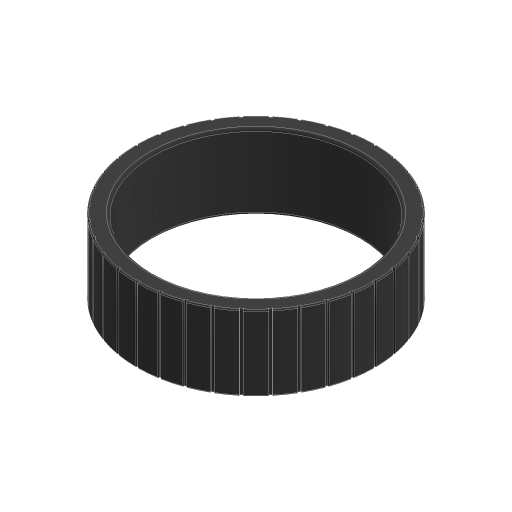
# Autodesk Inventor part: rubber
Saved by Autodesk Inventor 2023 (Build 270158000, 158)
## iProperties
Created: 2022-09-21
Part Number: rubber
Material: 고무
Document SubType Name: Modeling
Designer: doore
Density: 0.93 g/cm^3
Appearance: 고무 - 검은색
Author: doore
Autodesk Inventor part; units mm, degrees
ref_plane "YZ Plane" through (0, 0, 0) normal (1, 0, 0) x (0, 1, 0)
ref_plane "XZ Plane" through (0, 0, 0) normal (0, 1, 0) x (-1, 0, 0)
ref_plane "XY Plane" through (0, 0, 0) normal (0, 0, 1) x (1, 0, 0)
sketch "스케치1" plane through (0, 0, 0) normal (0, 1, 0) x (-1, 0, 0)
  circle A0 centre (0, 0) radius 27.5
  circle A1 centre (0, 0) radius 31.8
  line L0 (-31.25, -0.35) -> (-32.35, -0.35)
  line L1 (-32.35, -0.35) -> (-32.35, 0.35)
  line L2 (-32.35, 0.35) -> (-31.25, 0.35)
  line L3 (-31.25, 0.35) -> (-31.25, -0.35)
  circle A2 centre (0, 0) radius 31.8
  line L4 (-31.25, -0.35) -> (-32.35, 0.35) construction
  line L5 (-32.35, -0.35) -> (-31.25, 0.35) construction
  line L6 (-30.7145, -5.7712) -> (-31.7978, -5.9622)
  line L7 (-31.7978, -5.9622) -> (-31.9193, -5.2728)
  line L8 (-31.9193, -5.2728) -> (-30.836, -5.0818)
  line L9 (-30.836, -5.0818) -> (-30.7145, -5.7712)
  line L10 (-30.7145, -5.7712) -> (-31.9193, -5.2728) construction
  line L11 (-31.7978, -5.9622) -> (-30.836, -5.0818) construction
  line L12 (-29.2457, -11.017) -> (-30.2793, -11.3932)
  line L13 (-30.2793, -11.3932) -> (-30.5188, -10.7355)
  line L14 (-30.5188, -10.7355) -> (-29.4851, -10.3592)
  line L15 (-29.4851, -10.3592) -> (-29.2457, -11.017)
  line L16 (-29.2457, -11.017) -> (-30.5188, -10.7355) construction
  line L17 (-30.2793, -11.3932) -> (-29.4851, -10.3592) construction
  line L18 (-26.8883, -15.9281) -> (-27.8409, -16.4781)
  line L19 (-27.8409, -16.4781) -> (-28.1909, -15.8719)
  line L20 (-28.1909, -15.8719) -> (-27.2383, -15.3219)
  line L21 (-27.2383, -15.3219) -> (-26.8883, -15.9281)
  line L22 (-26.8883, -15.9281) -> (-28.1909, -15.8719) construction
  line L23 (-27.8409, -16.4781) -> (-27.2383, -15.3219) construction
  line L24 (-23.7139, -20.3552) -> (-24.5566, -21.0623)
  line L25 (-24.5566, -21.0623) -> (-25.0065, -20.5261)
  line L26 (-25.0065, -20.5261) -> (-24.1639, -19.819)
  line L27 (-24.1639, -19.819) -> (-23.7139, -20.3552)
  line L28 (-23.7139, -20.3552) -> (-25.0065, -20.5261) construction
  line L29 (-24.5566, -21.0623) -> (-24.1639, -19.819) construction
  line L30 (-19.819, -24.1639) -> (-20.5261, -25.0065)
  line L31 (-20.5261, -25.0065) -> (-21.0623, -24.5566)
  line L32 (-21.0623, -24.5566) -> (-20.3552, -23.7139)
  line L33 (-20.3552, -23.7139) -> (-19.819, -24.1639)
  line L34 (-19.819, -24.1639) -> (-21.0623, -24.5566) construction
  line L35 (-20.5261, -25.0065) -> (-20.3552, -23.7139) construction
  line L36 (-15.3219, -27.2383) -> (-15.8719, -28.1909)
  line L37 (-15.8719, -28.1909) -> (-16.4781, -27.8409)
  line L38 (-16.4781, -27.8409) -> (-15.9281, -26.8883)
  line L39 (-15.9281, -26.8883) -> (-15.3219, -27.2383)
  line L40 (-15.3219, -27.2383) -> (-16.4781, -27.8409) construction
  line L41 (-15.8719, -28.1909) -> (-15.9281, -26.8883) construction
  line L42 (-10.3592, -29.4851) -> (-10.7355, -30.5188)
  line L43 (-10.7355, -30.5188) -> (-11.3932, -30.2793)
  line L44 (-11.3932, -30.2793) -> (-11.017, -29.2457)
  line L45 (-11.017, -29.2457) -> (-10.3592, -29.4851)
  line L46 (-10.3592, -29.4851) -> (-11.3932, -30.2793) construction
  line L47 (-10.7355, -30.5188) -> (-11.017, -29.2457) construction
  line L48 (-5.0818, -30.836) -> (-5.2728, -31.9193)
  line L49 (-5.2728, -31.9193) -> (-5.9622, -31.7978)
  line L50 (-5.9622, -31.7978) -> (-5.7712, -30.7145)
  line L51 (-5.7712, -30.7145) -> (-5.0818, -30.836)
  line L52 (-5.0818, -30.836) -> (-5.9622, -31.7978) construction
  line L53 (-5.2728, -31.9193) -> (-5.7712, -30.7145) construction
  line L54 (0.35, -31.25) -> (0.35, -32.35)
  line L55 (0.35, -32.35) -> (-0.35, -32.35)
  line L56 (-0.35, -32.35) -> (-0.35, -31.25)
  line L57 (-0.35, -31.25) -> (0.35, -31.25)
  line L58 (0.35, -31.25) -> (-0.35, -32.35) construction
  line L59 (0.35, -32.35) -> (-0.35, -31.25) construction
  line L60 (5.7712, -30.7145) -> (5.9622, -31.7978)
  line L61 (5.9622, -31.7978) -> (5.2728, -31.9193)
  line L62 (5.2728, -31.9193) -> (5.0818, -30.836)
  line L63 (5.0818, -30.836) -> (5.7712, -30.7145)
  line L64 (5.7712, -30.7145) -> (5.2728, -31.9193) construction
  line L65 (5.9622, -31.7978) -> (5.0818, -30.836) construction
  line L66 (11.017, -29.2457) -> (11.3932, -30.2793)
  line L67 (11.3932, -30.2793) -> (10.7355, -30.5188)
  line L68 (10.7355, -30.5188) -> (10.3592, -29.4851)
  line L69 (10.3592, -29.4851) -> (11.017, -29.2457)
  line L70 (11.017, -29.2457) -> (10.7355, -30.5188) construction
  line L71 (11.3932, -30.2793) -> (10.3592, -29.4851) construction
  line L72 (15.9281, -26.8883) -> (16.4781, -27.8409)
  line L73 (16.4781, -27.8409) -> (15.8719, -28.1909)
  line L74 (15.8719, -28.1909) -> (15.3219, -27.2383)
  line L75 (15.3219, -27.2383) -> (15.9281, -26.8883)
  line L76 (15.9281, -26.8883) -> (15.8719, -28.1909) construction
  line L77 (16.4781, -27.8409) -> (15.3219, -27.2383) construction
  line L78 (20.3552, -23.7139) -> (21.0623, -24.5566)
  line L79 (21.0623, -24.5566) -> (20.5261, -25.0065)
  line L80 (20.5261, -25.0065) -> (19.819, -24.1639)
  line L81 (19.819, -24.1639) -> (20.3552, -23.7139)
  line L82 (20.3552, -23.7139) -> (20.5261, -25.0065) construction
  line L83 (21.0623, -24.5566) -> (19.819, -24.1639) construction
  line L84 (24.1639, -19.819) -> (25.0065, -20.5261)
  line L85 (25.0065, -20.5261) -> (24.5566, -21.0623)
  line L86 (24.5566, -21.0623) -> (23.7139, -20.3552)
  line L87 (23.7139, -20.3552) -> (24.1639, -19.819)
  line L88 (24.1639, -19.819) -> (24.5566, -21.0623) construction
  line L89 (25.0065, -20.5261) -> (23.7139, -20.3552) construction
  line L90 (27.2383, -15.3219) -> (28.1909, -15.8719)
  line L91 (28.1909, -15.8719) -> (27.8409, -16.4781)
  line L92 (27.8409, -16.4781) -> (26.8883, -15.9281)
  line L93 (26.8883, -15.9281) -> (27.2383, -15.3219)
  line L94 (27.2383, -15.3219) -> (27.8409, -16.4781) construction
  line L95 (28.1909, -15.8719) -> (26.8883, -15.9281) construction
  line L96 (29.4851, -10.3592) -> (30.5188, -10.7355)
  line L97 (30.5188, -10.7355) -> (30.2793, -11.3932)
  line L98 (30.2793, -11.3932) -> (29.2457, -11.017)
  line L99 (29.2457, -11.017) -> (29.4851, -10.3592)
  line L100 (29.4851, -10.3592) -> (30.2793, -11.3932) construction
  line L101 (30.5188, -10.7355) -> (29.2457, -11.017) construction
  line L102 (30.836, -5.0818) -> (31.9193, -5.2728)
  line L103 (31.9193, -5.2728) -> (31.7978, -5.9622)
  line L104 (31.7978, -5.9622) -> (30.7145, -5.7712)
  line L105 (30.7145, -5.7712) -> (30.836, -5.0818)
  line L106 (30.836, -5.0818) -> (31.7978, -5.9622) construction
  line L107 (31.9193, -5.2728) -> (30.7145, -5.7712) construction
  line L108 (31.25, 0.35) -> (32.35, 0.35)
  line L109 (32.35, 0.35) -> (32.35, -0.35)
  line L110 (32.35, -0.35) -> (31.25, -0.35)
  line L111 (31.25, -0.35) -> (31.25, 0.35)
  line L112 (31.25, 0.35) -> (32.35, -0.35) construction
  line L113 (32.35, 0.35) -> (31.25, -0.35) construction
  line L114 (30.7145, 5.7712) -> (31.7978, 5.9622)
  line L115 (31.7978, 5.9622) -> (31.9193, 5.2728)
  line L116 (31.9193, 5.2728) -> (30.836, 5.0818)
  line L117 (30.836, 5.0818) -> (30.7145, 5.7712)
  line L118 (30.7145, 5.7712) -> (31.9193, 5.2728) construction
  line L119 (31.7978, 5.9622) -> (30.836, 5.0818) construction
  line L120 (29.2457, 11.017) -> (30.2793, 11.3932)
  line L121 (30.2793, 11.3932) -> (30.5188, 10.7355)
  line L122 (30.5188, 10.7355) -> (29.4851, 10.3592)
  line L123 (29.4851, 10.3592) -> (29.2457, 11.017)
  line L124 (29.2457, 11.017) -> (30.5188, 10.7355) construction
  line L125 (30.2793, 11.3932) -> (29.4851, 10.3592) construction
  line L126 (26.8883, 15.9281) -> (27.8409, 16.4781)
  line L127 (27.8409, 16.4781) -> (28.1909, 15.8719)
  line L128 (28.1909, 15.8719) -> (27.2383, 15.3219)
  line L129 (27.2383, 15.3219) -> (26.8883, 15.9281)
  line L130 (26.8883, 15.9281) -> (28.1909, 15.8719) construction
  line L131 (27.8409, 16.4781) -> (27.2383, 15.3219) construction
  line L132 (23.7139, 20.3552) -> (24.5566, 21.0623)
  line L133 (24.5566, 21.0623) -> (25.0065, 20.5261)
  line L134 (25.0065, 20.5261) -> (24.1639, 19.819)
  line L135 (24.1639, 19.819) -> (23.7139, 20.3552)
  line L136 (23.7139, 20.3552) -> (25.0065, 20.5261) construction
  line L137 (24.5566, 21.0623) -> (24.1639, 19.819) construction
  line L138 (19.819, 24.1639) -> (20.5261, 25.0065)
  line L139 (20.5261, 25.0065) -> (21.0623, 24.5566)
  line L140 (21.0623, 24.5566) -> (20.3552, 23.7139)
  line L141 (20.3552, 23.7139) -> (19.819, 24.1639)
  line L142 (19.819, 24.1639) -> (21.0623, 24.5566) construction
  line L143 (20.5261, 25.0065) -> (20.3552, 23.7139) construction
  line L144 (15.3219, 27.2383) -> (15.8719, 28.1909)
  line L145 (15.8719, 28.1909) -> (16.4781, 27.8409)
  line L146 (16.4781, 27.8409) -> (15.9281, 26.8883)
  line L147 (15.9281, 26.8883) -> (15.3219, 27.2383)
  line L148 (15.3219, 27.2383) -> (16.4781, 27.8409) construction
  line L149 (15.8719, 28.1909) -> (15.9281, 26.8883) construction
  line L150 (10.3592, 29.4851) -> (10.7355, 30.5188)
  line L151 (10.7355, 30.5188) -> (11.3932, 30.2793)
  line L152 (11.3932, 30.2793) -> (11.017, 29.2457)
  line L153 (11.017, 29.2457) -> (10.3592, 29.4851)
  line L154 (10.3592, 29.4851) -> (11.3932, 30.2793) construction
  line L155 (10.7355, 30.5188) -> (11.017, 29.2457) construction
  line L156 (5.0818, 30.836) -> (5.2728, 31.9193)
  line L157 (5.2728, 31.9193) -> (5.9622, 31.7978)
  line L158 (5.9622, 31.7978) -> (5.7712, 30.7145)
  line L159 (5.7712, 30.7145) -> (5.0818, 30.836)
  line L160 (5.0818, 30.836) -> (5.9622, 31.7978) construction
  line L161 (5.2728, 31.9193) -> (5.7712, 30.7145) construction
  line L162 (-0.35, 31.25) -> (-0.35, 32.35)
  line L163 (-0.35, 32.35) -> (0.35, 32.35)
  line L164 (0.35, 32.35) -> (0.35, 31.25)
  line L165 (0.35, 31.25) -> (-0.35, 31.25)
  line L166 (-0.35, 31.25) -> (0.35, 32.35) construction
  line L167 (-0.35, 32.35) -> (0.35, 31.25) construction
  line L168 (-5.7712, 30.7145) -> (-5.9622, 31.7978)
  line L169 (-5.9622, 31.7978) -> (-5.2728, 31.9193)
  line L170 (-5.2728, 31.9193) -> (-5.0818, 30.836)
  line L171 (-5.0818, 30.836) -> (-5.7712, 30.7145)
  line L172 (-5.7712, 30.7145) -> (-5.2728, 31.9193) construction
  line L173 (-5.9622, 31.7978) -> (-5.0818, 30.836) construction
  line L174 (-11.017, 29.2457) -> (-11.3932, 30.2793)
  line L175 (-11.3932, 30.2793) -> (-10.7355, 30.5188)
  line L176 (-10.7355, 30.5188) -> (-10.3592, 29.4851)
  line L177 (-10.3592, 29.4851) -> (-11.017, 29.2457)
  line L178 (-11.017, 29.2457) -> (-10.7355, 30.5188) construction
  line L179 (-11.3932, 30.2793) -> (-10.3592, 29.4851) construction
  line L180 (-15.9281, 26.8883) -> (-16.4781, 27.8409)
  line L181 (-16.4781, 27.8409) -> (-15.8719, 28.1909)
  line L182 (-15.8719, 28.1909) -> (-15.3219, 27.2383)
  line L183 (-15.3219, 27.2383) -> (-15.9281, 26.8883)
  line L184 (-15.9281, 26.8883) -> (-15.8719, 28.1909) construction
  line L185 (-16.4781, 27.8409) -> (-15.3219, 27.2383) construction
  line L186 (-20.3552, 23.7139) -> (-21.0623, 24.5566)
  line L187 (-21.0623, 24.5566) -> (-20.5261, 25.0065)
  line L188 (-20.5261, 25.0065) -> (-19.819, 24.1639)
  line L189 (-19.819, 24.1639) -> (-20.3552, 23.7139)
  line L190 (-20.3552, 23.7139) -> (-20.5261, 25.0065) construction
  line L191 (-21.0623, 24.5566) -> (-19.819, 24.1639) construction
  line L192 (-24.1639, 19.819) -> (-25.0065, 20.5261)
  line L193 (-25.0065, 20.5261) -> (-24.5566, 21.0623)
  line L194 (-24.5566, 21.0623) -> (-23.7139, 20.3552)
  line L195 (-23.7139, 20.3552) -> (-24.1639, 19.819)
  line L196 (-24.1639, 19.819) -> (-24.5566, 21.0623) construction
  line L197 (-25.0065, 20.5261) -> (-23.7139, 20.3552) construction
  line L198 (-27.2383, 15.3219) -> (-28.1909, 15.8719)
  line L199 (-28.1909, 15.8719) -> (-27.8409, 16.4781)
  line L200 (-27.8409, 16.4781) -> (-26.8883, 15.9281)
  line L201 (-26.8883, 15.9281) -> (-27.2383, 15.3219)
  line L202 (-27.2383, 15.3219) -> (-27.8409, 16.4781) construction
  line L203 (-28.1909, 15.8719) -> (-26.8883, 15.9281) construction
  line L204 (-29.4851, 10.3592) -> (-30.5188, 10.7355)
  line L205 (-30.5188, 10.7355) -> (-30.2793, 11.3932)
  line L206 (-30.2793, 11.3932) -> (-29.2457, 11.017)
  line L207 (-29.2457, 11.017) -> (-29.4851, 10.3592)
  line L208 (-29.4851, 10.3592) -> (-30.2793, 11.3932) construction
  line L209 (-30.5188, 10.7355) -> (-29.2457, 11.017) construction
  line L210 (-30.836, 5.0818) -> (-31.9193, 5.2728)
  line L211 (-31.9193, 5.2728) -> (-31.7978, 5.9622)
  line L212 (-31.7978, 5.9622) -> (-30.7145, 5.7712)
  line L213 (-30.7145, 5.7712) -> (-30.836, 5.0818)
  line L214 (-30.836, 5.0818) -> (-31.7978, 5.9622) construction
  line L215 (-31.9193, 5.2728) -> (-30.7145, 5.7712) construction
  point P0 (-31.8, 0)
  point P1 (-31.3169, -5.522)
  point P2 (-29.8822, -10.8762)
  point P3 (-27.5396, -15.9)
  point P4 (-24.3602, -20.4406)
  point P5 (-20.4406, -24.3602)
  point P6 (-15.9, -27.5396)
  point P7 (-10.8762, -29.8822)
  point P8 (-5.522, -31.3169)
  point P9 (0, -31.8)
  point P10 (5.522, -31.3169)
  point P11 (10.8762, -29.8822)
  point P12 (15.9, -27.5396)
  point P13 (20.4406, -24.3602)
  point P14 (24.3602, -20.4406)
  point P15 (27.5396, -15.9)
  point P16 (29.8822, -10.8762)
  point P17 (31.3169, -5.522)
  point P18 (31.8, 0)
  point P19 (31.3169, 5.522)
  point P20 (29.8822, 10.8762)
  point P21 (27.5396, 15.9)
  point P22 (24.3602, 20.4406)
  point P23 (20.4406, 24.3602)
  point P24 (15.9, 27.5396)
  point P25 (10.8762, 29.8822)
  point P26 (5.522, 31.3169)
  point P27 (0, 31.8)
  point P28 (-5.522, 31.3169)
  point P29 (-10.8762, 29.8822)
  point P30 (-15.9, 27.5396)
  point P31 (-20.4406, 24.3602)
  point P32 (-24.3602, 20.4406)
  point P33 (-27.5396, 15.9)
  point P34 (-29.8822, 10.8762)
  point P35 (-31.3169, 5.522)
  point P36 (-31.7981, -0.35)
  point P37 (-31.3758, -5.177)
  point P38 (-31.2542, -5.8664)
  point P39 (-30.0001, -10.5467)
  point P40 (-29.7607, -11.2045)
  point P41 (-27.7129, -15.5959)
  point P42 (-27.3629, -16.2021)
  point P43 (-24.5837, -20.1713)
  point P44 (-24.1338, -20.7075)
  point P45 (-20.7075, -24.1338)
  point P46 (-20.1713, -24.5837)
  point P47 (-16.2021, -27.3629)
  point P48 (-15.5959, -27.7129)
  point P49 (-11.2045, -29.7607)
  point P50 (-10.5467, -30.0001)
  point P51 (-5.8664, -31.2542)
  point P52 (-5.177, -31.3758)
  point P53 (-0.35, -31.7981)
  point P54 (0.35, -31.7981)
  point P55 (5.177, -31.3758)
  point P56 (5.8664, -31.2542)
  point P57 (10.5467, -30.0001)
  point P58 (11.2045, -29.7607)
  point P59 (15.5959, -27.7129)
  point P60 (16.2021, -27.3629)
  point P61 (20.1713, -24.5837)
  point P62 (20.7075, -24.1338)
  point P63 (24.1338, -20.7075)
  point P64 (24.5837, -20.1713)
  point P65 (27.3629, -16.2021)
  point P66 (27.7129, -15.5959)
  point P67 (29.7607, -11.2045)
  point P68 (30.0001, -10.5467)
  point P69 (31.2542, -5.8664)
  point P70 (31.3758, -5.177)
  point P71 (31.7981, -0.35)
  point P72 (31.7981, 0.35)
  point P73 (31.3758, 5.177)
  point P74 (31.2542, 5.8664)
  point P75 (30.0001, 10.5467)
  point P76 (29.7607, 11.2045)
  point P77 (27.7129, 15.5959)
  point P78 (27.3629, 16.2021)
  point P79 (24.5837, 20.1713)
  point P80 (24.1338, 20.7075)
  point P81 (20.7075, 24.1338)
  point P82 (20.1713, 24.5837)
  point P83 (16.2021, 27.3629)
  point P84 (15.5959, 27.7129)
  point P85 (11.2045, 29.7607)
  point P86 (10.5467, 30.0001)
  point P87 (5.8664, 31.2542)
  point P88 (5.177, 31.3758)
  point P89 (0.35, 31.7981)
  point P90 (-0.35, 31.7981)
  point P91 (-5.177, 31.3758)
  point P92 (-5.8664, 31.2542)
  point P93 (-10.5467, 30.0001)
  point P94 (-11.2045, 29.7607)
  point P95 (-15.5959, 27.7129)
  point P96 (-16.2021, 27.3629)
  point P97 (-20.1713, 24.5837)
  point P98 (-20.7075, 24.1338)
  point P99 (-24.1338, 20.7075)
  point P100 (-24.5837, 20.1713)
  point P101 (-27.3629, 16.2021)
  point P102 (-27.7129, 15.5959)
  point P103 (-29.7607, 11.2045)
  point P104 (-30.0001, 10.5467)
  point P105 (-31.2542, 5.8664)
  point P106 (-31.3758, 5.177)
  point P107 (-31.7981, 0.35)
  dimension "d0" = 55
  dimension "d1" = 4.3
  dimension "d13" = 1.1
  dimension "d14" = 0.7
  dimension "d15" = 360
  constraints: 432 end point, 2 midpoint, 2 parallel, 1 centre point, 1 coincident, 1 horizontal, 1 horizontal alignment, 1 perpendicular, 401 other
  measures "d0" diameter of A0
  measures "d13" distance of L1.end L2.end
  measures "d14" distance of L0.end L1.end
extrude "돌출2" add sketch "스케치1" along normal blind 20 contours L108 L111 L110 A1 L102 L105 L104 L96 L99 L98 L90 L93 L92 L84 L87 L86 L78 L81 L80 L72 L75 L74 L66 L69 L68 L60 L63 L62 L54 L57 L56 L48 L51 L50 L42 L45 L44 L36 L39 L38 L30 L33 L32 L24 L27 L26 L18 L21 L20 L12 L15 L14 L6 L9 L8 L0 L3 L2 L210 L213 L212 L204 L207 L206 L198 L201 L200 L192 L195 L194 L186 L189 L188 L180 L183 L182 L174 L177 L176 L168 L171 L170 L162 L165 L164 L156 L159 L158 L150 L153 L152 L144 L147 L146 L138 L141 L140 L132 L135 L134 L126 L129 L128 L120 L123 L122 L114 L117 L116
fillet "모깎기2" radius 0.7 2 edges at (27.5, 20, 0) (27.5, 0, 0)
fillet "모깎기3" radius 0.3 36 edges at (-31.679, 20, -2.7716) (-31.679, 20, 2.7716) (-30.7164, 20, 8.2304) (-28.8206, 20, 13.4393) (-26.049, 20, 18.2397) (-22.486, 20, 22.486) (-18.2397, 20, 26.049) (-13.4393, 20, 28.8206) (-8.2304, 20, 30.7164) (-2.7716, 20, 31.679) (2.7716, 20, 31.679) (8.2304, 20, 30.7164) (13.4393, 20, 28.8206) (18.2397, 20, 26.049) (22.486, 20, 22.486) (26.049, 20, 18.2397) (28.8206, 20, 13.4393) (30.7164, 20, 8.2304) (31.679, 20, 2.7716) (31.679, 20, -2.7716) (30.7164, 20, -8.2304) (28.8206, 20, -13.4393) (26.049, 20, -18.2397) (22.486, 20, -22.486) (18.2397, 20, -26.049) (13.4393, 20, -28.8206) (8.2304, 20, -30.7164) (2.7716, 20, -31.679) (-2.7716, 20, -31.679) (-8.2304, 20, -30.7164) (-13.4393, 20, -28.8206) (-18.2397, 20, -26.049) (-22.486, 20, -22.486) (-26.049, 20, -18.2397) (-28.8206, 20, -13.4393) (-30.7164, 20, -8.2304)
fillet "모깎기4" radius 0.3 36 edges at (2.7716, 0, -31.679) (-2.7716, 0, -31.679) (-8.2304, 0, -30.7164) (-13.4393, 0, -28.8206) (-18.2397, 0, -26.049) (-22.486, 0, -22.486) (-26.049, 0, -18.2397) (-28.8206, 0, -13.4393) (-30.7164, 0, -8.2304) (-31.679, 0, -2.7716) (-31.679, 0, 2.7716) (-30.7164, 0, 8.2304) (-28.8206, 0, 13.4393) (-26.049, 0, 18.2397) (-22.486, 0, 22.486) (-18.2397, 0, 26.049) (-13.4393, 0, 28.8206) (-8.2304, 0, 30.7164) (-2.7716, 0, 31.679) (2.7716, 0, 31.679) (8.2304, 0, 30.7164) (13.4393, 0, 28.8206) (18.2397, 0, 26.049) (22.486, 0, 22.486) (26.049, 0, 18.2397) (28.8206, 0, 13.4393) (30.7164, 0, 8.2304) (31.679, 0, 2.7716) (31.679, 0, -2.7716) (30.7164, 0, -8.2304) (28.8206, 0, -13.4393) (26.049, 0, -18.2397) (22.486, 0, -22.486) (18.2397, 0, -26.049) (13.4393, 0, -28.8206) (8.2304, 0, -30.7164)
